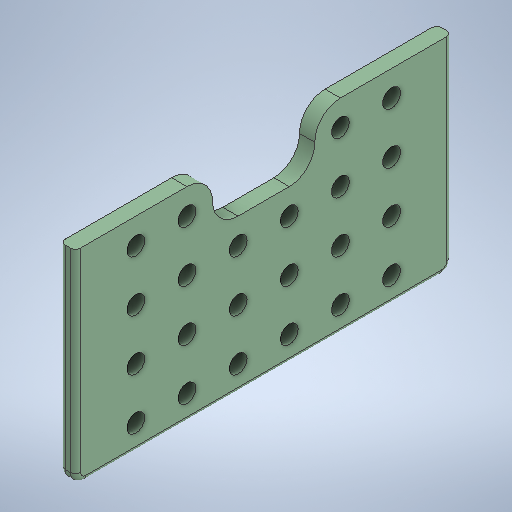
# Autodesk Inventor part: plaque
Saved by Autodesk Inventor 2025 (Build 290162000, 162)
## iProperties
Created: 2024-09-05
Part Number: plaque
Material: Générique
Document SubType Name: Modeling
Designer: chass
Density: 1 g/cm^3
Appearance: Par défaut
Author: chass
Autodesk Inventor part; units mm, degrees
ref_plane "YZ Plane" through (0, 0, 0) normal (1, 0, 0) x (0, 1, 0)
ref_plane "XZ Plane" through (0, 0, 0) normal (0, 1, 0) x (-1, 0, 0)
ref_plane "XY Plane" through (0, 0, 0) normal (0, 0, 1) x (1, 0, 0)
sketch "Esquisse1" plane through (0, 0, 0) normal (0, 1, 0) x (-1, 0, 0)
  line L0 (1.5706, 65.8) -> (-1.4294, 65.8)
  line L1 (-1.4294, 65.8) -> (-1.4294, -7.8)
  line L2 (-1.4294, -7.8) -> (1.5706, -7.8)
  line L3 (1.5706, -7.8) -> (1.5706, 65.8)
  point P0 (0, 0)
  dimension "d0" = 3
  dimension "d1" = 73.6
  constraints: 8 end point, 2 parallel, 1 horizontal, 1 perpendicular
  measures "d0" distance of L1.end L2.end
  measures "d1" distance of L2.end L0.start
extrude "Extrusion1" add sketch "Esquisse1" along normal blind 40
fillet "Congé1" radius 2 2 edges at (-0.0706, 0, 65.8) (-0.0706, 0, -7.8)
fillet "Congé2" radius 1 10 edges at (1.4294, 0.5858, -7.2142) (1.4294, 21, -7.8) (1.4294, 0.5858, 65.2142) (1.4294, 21, 65.8) (1.4294, 0, 29) (-1.5706, 0.5858, 65.2142) (-1.5706, 21, 65.8) (-1.5706, 0.5858, -7.2142) (-1.5706, 21, -7.8) (-1.5706, 0, 29)
sketch "Esquisse2" plane through (1.4294, 2, -6.8) normal (1, 0, 0) x (0, 0, -1)
  line L0 (-72.6, 38) -> (1, 38)
  line L1 (1, 38) -> (1, -2)
  line L2 (1, -2) -> (-72.6, -2)
  line L3 (-72.6, -2) -> (-72.6, 38)
  line L4 (-35.8, 38) -> (-35.8, -2)
  line L5 (-72.6, 18) -> (1, 18)
  circle A0 centre (-40.8, 23) radius 1.75
  circle A1 centre (-50.8, 23) radius 1.75
  circle A2 centre (-60.8, 23) radius 1.75
  circle A3 centre (-60.8, 33) radius 1.75
  circle A4 centre (-50.8, 33) radius 1.75
  circle A5 centre (-40.8, 13) radius 1.75
  circle A6 centre (-50.8, 13) radius 1.75
  circle A7 centre (-60.8, 13) radius 1.75
  circle A8 centre (-60.8, 3) radius 1.75
  circle A9 centre (-50.8, 3) radius 1.75
  circle A10 centre (-40.8, 3) radius 1.75
  circle A11 centre (-30.8, 23) radius 1.75
  circle A12 centre (-20.8, 23) radius 1.75
  circle A13 centre (-10.8, 23) radius 1.75
  circle A14 centre (-10.8, 33) radius 1.75
  circle A15 centre (-20.8, 33) radius 1.75
  circle A16 centre (-30.8, 13) radius 1.75
  circle A17 centre (-30.8, 3) radius 1.75
  circle A18 centre (-20.8, 13) radius 1.75
  circle A19 centre (-20.8, 3) radius 1.75
  circle A20 centre (-10.8, 3) radius 1.75
  circle A21 centre (-10.8, 13) radius 1.75
  line L6 (-45.8, 38) -> (-45.8, 28)
  line L7 (-45.8, 28) -> (-25.8, 28)
  line L8 (-25.8, 28) -> (-25.8, 38)
  line L9 (-25.8, 38) -> (-45.8, 38)
  point P0 (-6.8, -2)
  point P1 (-45.8, 38)
  dimension "d6" = 3.5
  dimension "d7" = 3.5
  dimension "d8" = 3.5
  dimension "d10" = 5
  dimension "d11" = 10
  dimension "d12" = 10
  dimension "d14" = 3.5
  dimension "d15" = 10
  dimension "d16" = 3.5
  dimension "d17" = 10
  dimension "d21" = 5
  dimension "d24" = 10
  dimension "d26" = 20
  dimension "d27" = 10
  dimension "d28" = 36.8
  constraints: 22 centre point, 20 end point, 16 symmetric about line, 4 midpoint, 2 parallel, 2 perpendicular, 1 collinear, 1 horizontal, 1 vertical, 16 other
  measures "d6" diameter of A0
  measures "d7" diameter of A1
  measures "d8" diameter of A2
  measures "d10" distance from line of L4 A0.centre
  measures "d11" distance of A1.centre A0.centre
  measures "d12" distance of A2.centre A1.centre
  measures "d14" diameter of A3
  measures "d15" distance of A3.centre A2.centre
  measures "d16" diameter of A4
  measures "d17" distance of A4.centre A1.centre
  measures "d21" distance from line of L5 A0.centre
  measures "d24" distance of L7.end L8.end
  measures "d26" distance of L6.end L7.end
  measures "d27" distance between parallel lines of L8 L4
  measures "d28" distance between parallel lines of L1 L4
extrude "Extrusion2" cut sketch "Esquisse2" against normal blind 40 contours L0 L4 L7 L6 | L0 L8 L7 L4 | A0 | A1 | A2 | A3 | A4 | A5 | A6 | A7 | A8 | A9 | A10 | A11 | A12 | A13 | A14 | A15 | A16 | A17 | A18 | A19 | A20 | A21
fillet "Congé3" radius 5 4 edges at (-0.0706, 30, 19) (-0.0706, 30, 39) (-0.0706, 40, 19) (-0.0706, 40, 39)
